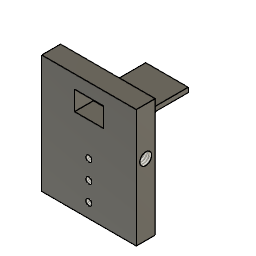
XY Plotter Left Edge (Autodesk Fusion 360 design; units mm, degrees)
Autodesk Fusion 360 part; units mm, degrees
note: some values were not read from the file. Chosen so that the rebuilt part matches the saved one: which bodies a step acts on.
sketch "Sketch1" plane through (0, 0, 0) normal (0, 1, 0) x (1, 0, 0)
  line L0 (-6.1, -4.1) -> (6.1, -4.1)
  line L1 (6.1, -4.1) -> (6.1, 4.1)
  line L2 (6.1, 4.1) -> (-6.1, 4.1)
  line L3 (-6.1, 4.1) -> (-6.1, -4.1)
  line L4 (-6.1, -4.1) -> (6.1, 4.1) construction
  line L5 (6.1, -4.1) -> (-6.1, 4.1) construction
  line L6 (-20, -9.7099) -> (20, -9.7099)
  line L7 (20, -9.7099) -> (20, 40.2901)
  line L8 (20, 40.2901) -> (-20, 40.2901)
  line L9 (-20, 40.2901) -> (-20, -9.7099)
  point P0 (-0.0519, 34.2901)
  point P1 (-0.0519, 26.2901)
  point P2 (-0.0519, 18.2901)
  dimension "d1" = 12.2
  dimension "d2" = 8.2
  dimension "d3" = 40
  dimension "d4" = 50
  dimension "d8" = 20
  dimension "d30" = 6
  dimension "d31" = 8
  dimension "d32" = 8
  dimension "d33" = 36.1901
  constraint horizontal L0
  constraint perpendicular L0 L1
  constraint parallel L0 L2
  constraint parallel L1 L3
  constraint coincident L4 origin
  constraint coincident L5 origin
  constraint horizontal L6
  constraint vertical L7
  constraint horizontal L8
  constraint vertical L9
  measures "d1" distance of L1.end L2.end
  measures "d2" distance of L0.end L1.end
  measures "d3" distance of L6.start L6.end
  measures "d4" distance of L6.start L8.end
  measures "d8" distance of origin L9
  measures "d30" distance of L8 P0
  measures "d31" distance of P0 P1
  measures "d32" distance of P1 P2
  measures "d33" distance of L2 L8
sketch "Sketch2" plane through (0, 0, 0) normal (1, 0, 0) x (0, 1, 0)
  line L0 (0, 0) -> (0, -4.1) construction
  line L1 (0, -4.1) -> (25, -4.1)
  line L2 (25, -4.1) -> (25, -6.1)
  line L3 (25, -6.1) -> (0, -6.1)
  line L4 (0, -6.1) -> (0, -4.1)
  line L5 (0, -6.1) -> (0, -12.1)
  line L6 (0, -12.1) -> (4, -12.1)
  line L7 (0, -6.1) -> (8, -6.1)
  line L8 (8, -6.1) -> (8, -8.1)
  line L9 (8, -8.1) -> (4, -12.1)
  dimension "d9" = 4.1
  dimension "d10" = 25
  dimension "d11" = 2
  dimension "d12" = 6
  dimension "d13" = 4
  dimension "d14" = 8
  dimension "d15" = 2
  constraint coincident L0.start origin
  constraint vertical L0
  constraint horizontal L1
  constraint vertical L2
  constraint horizontal L3
  constraint vertical L4
  constraint perpendicular L3 L5
  constraint perpendicular L5 L6
  constraint perpendicular L5 L7
  constraint perpendicular L7 L8
  measures "d9" distance of L0.start L0.end
  measures "d10" distance of L0.end L1.end
  measures "d11" distance of L0.end L3.end
  measures "d12" distance of L3.end L5.end
  measures "d13" distance of L5.end L6.end
  measures "d14" distance of L3.end L7.end
  measures "d15" distance of L7.end L8.end
extrude "Extrude1" add sketch "Sketch1" against normal blind 8 makes body 1
extrude "Extrude2" add sketch "Sketch2" along normal mid plane 18 separate body contours L1 L2 L3 L4 L7 makes body 2
extrude "Extrude3" add sketch "Sketch2" along normal mid plane 18 separate body contours L3 L5 L6 L7 L8 L9 makes body 3
extrude "Extrude4" cut sketch "Sketch2" along normal mid plane 14 contours L3 L5 L6 L7 L8 L9 bodies 1 2 3 makes body 4 at (7, 4, -8.7667)
sketch "Sketch4" plane through (0, 0, -4.1) normal (0, 0, 1) x (-1, 0, 0)
  line L0 (9, 0) -> (-9, 0)
  line L1 (-9, 0) -> (-9, -25)
  line L2 (-9, -25) -> (9, -25)
  line L3 (9, -25) -> (9, 0)
  point P0 (0, -8.5)
  dimension "d24" = 8.5
  measures "d24" distance of L0 P0
hole "Hole1" at (0, 8.5, -4.1) direction (0, 0, -1) diameter 2.529 depth 20 tip angle 118 bodies 2
thread "Thread1" "ISO Metric profile 3.0 M3x0.5 M3x0.5 6H" thread offset 0 thread depth 7.4
hole "Hole2" at (-0.0519, 0, -18.2901) at (-0.0519, 0, -26.2901) at (-0.0519, 0, -34.2901) direction (0, -1, 0) diameter 2.529 depth 20 tip angle 118 bodies 1
thread "Thread2" "ISO Metric profile 3.0 M3x0.5 M3x0.5 6H" thread offset 0 thread depth 7.4
ref_plane "WorkPlane1" through (0, -4, -15.2901) normal (0, -1, 0) x (0, 0, -1)
sketch "Sketch5" plane through (0, -4, 0) normal (0, -1, 0) x (-1, 0, 0)
  line L0 (-2.9571, 15.8994) -> (2.7106, 15.8994)
  line L1 (2.7106, 15.8994) -> (2.7106, 37.2255)
  line L2 (2.7106, 37.2255) -> (-2.9571, 37.2255)
  line L3 (-2.9571, 37.2255) -> (-2.9571, 15.8994)
  constraint horizontal L0
  constraint vertical L1
  constraint horizontal L2
  constraint vertical L3
extrude "Extrude5" add sketch "Sketch5" along normal mid plane 2 separate body makes body 5
sketch "Sketch6" plane through (20, 0, 0) normal (1, 0, 0) x (0, 1, 0)
  line L0 (0, -40.2901) -> (0, 9.7099)
  line L1 (0, 9.7099) -> (-8, 9.7099)
  line L2 (-8, 9.7099) -> (-8, -40.2901)
  line L3 (-8, -40.2901) -> (0, -40.2901)
  circle A0 centre (-4, -10.2901) radius 3
  point P0 (-4, -10.2901)
  dimension "d41" = 20
  dimension "d48" = 6
  constraint coincident P0 A0.centre
  measures "d41" distance of L1 P0
  measures "d48" diameter of A0
hole "Hole3" at (20, -4, -10.2901) direction (-1, 0, 0) diameter 5.035 depth 20 tip angle 118 bodies 1
thread "Thread3" "ISO Metric profile 6.0 M6x1 M6x1 6H" thread offset 0 thread depth 7.4
